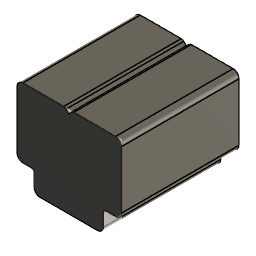
Conector (Autodesk Fusion 360 design; units mm, degrees)
part number: 2025-12-28-14-48-56-748
Autodesk Fusion 360 part; units mm, degrees
sketch "Boceto1" plane through (0, 0, 0) normal (0, 1, 0) x (1, 0, 0)
  line L0 (1.95, 0) -> (6.85, 0)
  line L1 (8.89, -2.3) -> (8.89, -7.2)
  line L2 (0, -7.2) -> (0, -2.3)
  line L3 (1.45, -0.5) -> (1.45, -1.6)
  line L4 (1.25, -1.8) -> (0.5, -1.8)
  line L5 (7.35, -0.5) -> (7.35, -1.6)
  line L6 (7.55, -1.8) -> (8.39, -1.8)
  arc A0 (0, -7.2) -> (0.5, -7.7) centre (0.5, -7.2) ccw
  arc A1 (8.39, -7.7) -> (8.89, -7.2) centre (8.39, -7.2) ccw
  arc A2 (8.89, -2.3) -> (8.39, -1.8) centre (8.39, -2.3) ccw
  arc A3 (0.5, -1.8) -> (0, -2.3) centre (0.5, -2.3) ccw
  arc A4 (1.95, 0) -> (1.45, -0.5) centre (1.95, -0.5) ccw
  arc A5 (7.35, -0.5) -> (6.85, 0) centre (6.85, -0.5) ccw
  arc A6 (1.25, -1.8) -> (1.45, -1.6) centre (1.25, -1.6) ccw
  arc A7 (7.35, -1.6) -> (7.55, -1.8) centre (7.55, -1.6) ccw
  line L7 (4.1882, -7.6102) -> (4.425, -7.3692)
  line L8 (4.425, -7.3692) -> (4.61, -7.5918)
  line L9 (0.5, -7.7) -> (3.9742, -7.7)
  line L10 (4.8407, -7.7) -> (8.39, -7.7)
  arc A8 (3.9742, -7.7) -> (4.1882, -7.6102) centre (3.9742, -7.4) ccw
  arc A9 (4.61, -7.5918) -> (4.8407, -7.7) centre (4.8407, -7.4) ccw
  point P0 (0, -7.7)
  dimension "d1" = 7.7
  dimension "d3" = 0.5
  dimension "d4" = 0.2
  dimension "d5" = 0.3
  constraint horizontal L0
  constraint vertical L1
  constraint vertical L2
  constraint vertical L3
  constraint horizontal L4
  constraint vertical L5
  constraint horizontal L6
  constraint coincident P0 L2
  constraint tangent L2 A0
  constraint tangent L1 A1
  constraint equal A0 A1
  constraint tangent L6 A2
  constraint tangent L1 A2
  constraint equal A0 A2
  constraint tangent L4 A3
  constraint tangent L2 A3
  constraint equal A0 A3
  constraint tangent L3 A4
  constraint tangent L0 A4
  constraint equal A0 A4
  constraint tangent L5 A5
  constraint tangent L0 A5
  constraint equal A0 A5
  constraint tangent L3 A6
  constraint tangent L4 A6
  constraint tangent L5 A7
  constraint tangent L6 A7
  constraint equal A6 A7
  constraint tangent A1 L10
  constraint tangent L7 A8
  constraint tangent L9 A8
  constraint tangent L8 A9
  constraint tangent L10 A9
  constraint equal A8 A9
  measures "d1" distance of origin P0
  measures "d3" radius of A0
  measures "d4" radius of A6
  measures "d5" radius of A8
extrude "Extruir1" add sketch "Boceto1" along normal blind 10
equation "L = 10 mm"
equation "d7 = L"
